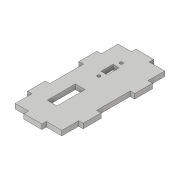
# Autodesk Inventor part: costat4
Saved by Autodesk Inventor 2019 (Build 230136000, 136)
## iProperties
Created: 2018-09-21
Part Number: costat4
Material: Genérico
Document SubType Name: Modeling
Designer: lmacia
Density: 1 g/cm^3
Appearance: Valor por defecto
Author: lmacia
Autodesk Inventor part; units mm, degrees
ref_plane "YZ Plane" through (0, 0, 0) normal (1, 0, 0) x (0, 1, 0)
ref_plane "XZ Plane" through (0, 0, 0) normal (0, 1, 0) x (-1, 0, 0)
ref_plane "XY Plane" through (0, 0, 0) normal (0, 0, 1) x (1, 0, 0)
sketch "Boceto1" plane through (0, 0, 0) normal (0, 1, 0) x (-1, 0, 0)
  line L0 (-11.7171, -8.4187) -> (-13.9671, -8.4187)
  line L1 (-13.9671, -8.4187) -> (-13.9671, -17.4187)
  line L2 (-13.9671, -17.4187) -> (-11.7171, -17.4187)
  line L3 (-11.7171, -17.4187) -> (-11.7171, -25.8375)
  line L4 (-11.7171, -25.8375) -> (-3.9546, -25.8375)
  line L5 (-3.9546, -25.8375) -> (-3.9546, -28.0875)
  line L6 (-3.9546, -28.0875) -> (5.0454, -28.0875)
  line L7 (5.0454, -28.0875) -> (5.0454, -25.8375)
  line L8 (5.0454, -25.8375) -> (11.6829, -25.8375)
  line L9 (11.6829, -25.8375) -> (11.6829, -17.4194)
  line L10 (11.6829, -17.4194) -> (13.9329, -17.4187)
  line L11 (13.9329, -17.4187) -> (13.9329, -8.4187)
  line L12 (13.9329, -8.4187) -> (11.6829, -8.4187)
  line L13 (11.6829, -8.4187) -> (11.6829, 8.4188)
  line L14 (11.6829, 8.4188) -> (13.9329, 8.4188)
  line L15 (13.9329, 8.4188) -> (13.9329, 17.4188)
  line L16 (13.9329, 17.4188) -> (11.6829, 17.4188)
  line L17 (11.6829, 17.4188) -> (11.6829, 21.3375)
  line L18 (11.6829, 21.3375) -> (11.6829, 25.8375)
  line L19 (11.6829, 25.8375) -> (5.0454, 25.8375)
  line L20 (5.0454, 25.8375) -> (5.0454, 28.0875)
  line L21 (5.0454, 28.0875) -> (-3.9546, 28.0875)
  line L22 (-3.9546, 28.0875) -> (-3.9546, 25.8375)
  line L23 (-3.9546, 25.8375) -> (-10.5921, 25.8375)
  line L24 (-10.5921, 25.8375) -> (-10.9671, 25.8375)
  line L25 (-10.9671, 25.8375) -> (-11.7171, 25.8375)
  line L26 (-11.7171, 25.8375) -> (-11.7171, 17.4188)
  line L27 (-11.7171, 17.4188) -> (-13.9671, 17.4188)
  line L28 (-13.9671, 17.4188) -> (-13.9671, 8.4188)
  line L29 (-13.9671, 8.4188) -> (-11.7171, 8.4188)
  line L30 (-11.7171, 8.4188) -> (-11.7171, -8.4187)
  line L31 (4.1079, -15.7125) -> (1.1079, -15.7125)
  line L32 (1.1079, -15.7125) -> (1.1079, -9.7125)
  line L33 (1.1079, -9.7125) -> (4.1079, -9.7125)
  line L34 (4.1079, -9.7125) -> (4.1079, -15.7125)
  line L35 (0.1704, 2.2875) -> (0.1704, 16.3875)
  line L36 (0.1704, 16.3875) -> (5.0454, 16.3875)
  line L37 (5.0454, 16.3875) -> (5.0454, 2.2875)
  line L38 (5.0454, 2.2875) -> (0.1704, 2.2875)
  circle A0 centre (2.6079, -7.0875) radius 0.75
  circle A1 centre (2.6079, -18.3375) radius 0.75
  point P0 (0, 0)
  constraints: 78 end point, 2 centre point
extrude "Extrusión1" add sketch "Boceto1" along normal blind 2.4
